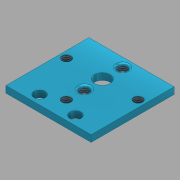
# Autodesk Inventor part: DC Motor-25 Bracket B-Blue
Saved by Autodesk Inventor 2017 (Build 210142000, 142)
## iProperties
Created: 2017-05-07
Part Number: DC Motor-25 Bracket B-Blue
Material: Aluminum 6061
Document SubType Name: Modeling
Designer: zallen
Density: 2.7 g/cm^3
Appearance: Makeblock Blue
Mass: 10.2499 g
Surface Area: 33.2954 cm^2
Volume: 3.79624 cm^3
Catalog Web Link: http://www.makeblock.com/dc-motor-25-bracket-b-blue-pair
Author: zallen
Autodesk Inventor part; units mm, degrees
ref_plane "YZ Plane" through (0, 0, 0) normal (1, 0, 0) x (0, 1, 0)
ref_plane "XZ Plane" through (0, 0, 0) normal (0, 1, 0) x (-1, 0, 0)
ref_plane "XY Plane" through (0, 0, 0) normal (0, 0, 1) x (1, 0, 0)
sketch "Sketch1" plane through (0, 0, 0) normal (0, 0, 1) x (1, 0, 0)
  line L0 (0, 0) -> (38, 0)
  line L1 (38, 0) -> (38, 37)
  line L2 (38, 37) -> (0, 37)
  line L3 (0, 37) -> (0, 0)
  line L4 (19, 37) -> (19, 0) construction
  circle A0 centre (11, 4) radius 2.5
  circle A1 centre (27, 4) radius 2.5
  circle A2 centre (19, 8) radius 2
  circle A3 centre (19, 16) radius 2
  circle A4 centre (19, 24) radius 3.5
  circle A5 centre (19, 33) radius 2
  circle A6 centre (3, 24) radius 2
  circle A7 centre (35, 24) radius 2
  dimension "d0" = 38
  dimension "d1" = 37
  dimension "d2" = 5
  dimension "d3" = 8
  dimension "d4" = 4
  dimension "d5" = 5
  dimension "d6" = 8
  dimension "d7" = 4
  dimension "d8" = 4
  dimension "d9" = 8
  dimension "d10" = 4
  dimension "d11" = 16
  dimension "d12" = 7
  dimension "d13" = 24
  dimension "d14" = 4
  dimension "d15" = 17
  dimension "d18" = 4
  dimension "d19" = 4
  dimension "d20" = 32
  dimension "d21" = 3
  dimension "d22" = 13
  dimension "d23" = 13
  constraints: 10 end point, 8 centre point, 4 point on line, 2 midpoint, 2 parallel, 1 horizontal, 1 perpendicular
  measures "d0" distance of L1.end L2.end
  measures "d1" distance of L0.end L1.end
  measures "d2" diameter of A0
  measures "d3" distance from line of A0.centre L4
  measures "d4" distance from line of L0 A0.centre
  measures "d5" diameter of A1
  measures "d6" distance from line of L4 A1.centre
  measures "d7" distance from line of L0 A1.centre
  measures "d8" diameter of A2
  measures "d9" distance from line of L0 A2.centre
  measures "d10" diameter of A3
  measures "d11" distance from line of L0 A3.centre
  measures "d12" diameter of A4
  measures "d13" distance from line of L0 A4.centre
  measures "d14" diameter of A5
  measures "d15" distance of A3.centre A5.centre
  measures "d18" diameter of A6
  measures "d19" diameter of A7
  measures "d20" distance of A7.centre A6.centre
  measures "d21" distance from line of L3 A6.centre
  measures "d22" distance from line of L2 A6.centre
  measures "d23" distance from line of L2 A7.centre
extrude "Extrusion1" add sketch "Sketch1" along normal blind 3
thread "Thread1" size "M4x0.7" class "6H" standard "ISO Metric profile" full length
thread "Thread2" size "M4x0.7" class "6H" standard "ISO Metric profile" full length
thread "Thread3" size "M4x0.7" class "6H" standard "ISO Metric profile" full length
thread "Thread4" size "M4x0.7" class "6H" standard "ISO Metric profile" full length
thread "Thread5" size "M4x0.7" class "6H" standard "ISO Metric profile" full length
fillet "Fillet1" radius 1 2 edges at (17, 33, 3) (17, 16, 3)
body "Solid1"
